Autodesk Inventor part; units mm, degrees
(part 2 of 3)
  line L1031 (-10.05, 26.35) -> (-10.15, 26.35)
  line L1032 (-10.15, 26.35) -> (-10.15, 26.05)
  line L1033 (-10.05, 26.05) -> (-10.05, 26.35)
  line L1034 (-9.175, 25.6738) -> (-9.175, 25.9738)
  line L1035 (-9.275, 25.9738) -> (-9.275, 25.6738)
  line L1036 (-9.275, 25.6738) -> (-9.175, 25.6738)
  line L1037 (-9.425, 25.6738) -> (-9.425, 25.9738)
  line L1038 (-9.525, 25.9738) -> (-9.525, 25.6738)
  line L1039 (-9.525, 25.6738) -> (-9.425, 25.6738)
  line L1040 (-9.425, 25.9738) -> (-9.525, 25.9738)
  line L1041 (-9.175, 25.9738) -> (-9.275, 25.9738)
  line L1042 (-8.675, 25.6738) -> (-8.675, 25.9738)
  line L1043 (-8.775, 25.9738) -> (-8.775, 25.6738)
  line L1044 (-8.675, 25.9738) -> (-8.775, 25.9738)
  line L1045 (-8.775, 25.6738) -> (-8.675, 25.6738)
  line L1046 (-8.925, 25.6738) -> (-8.925, 25.9738)
  line L1047 (-8.925, 25.9738) -> (-9.025, 25.9738)
  line L1048 (-9.025, 25.9738) -> (-9.025, 25.6738)
  line L1049 (-9.025, 25.6738) -> (-8.925, 25.6738)
  line L1050 (-8.175, 25.9738) -> (-8.275, 25.9738)
  line L1051 (-8.425, 25.9738) -> (-8.525, 25.9738)
  line L1052 (-8.175, 25.6738) -> (-8.175, 25.9738)
  line L1053 (-8.275, 25.9738) -> (-8.275, 25.6738)
  line L1054 (-8.275, 25.6738) -> (-8.175, 25.6738)
  line L1055 (-8.425, 25.6738) -> (-8.425, 25.9738)
  line L1056 (-8.525, 25.9738) -> (-8.525, 25.6738)
  line L1057 (-8.525, 25.6738) -> (-8.425, 25.6738)
  line L1058 (-7.775, 25.9738) -> (-7.775, 25.6738)
  line L1059 (-7.675, 25.9738) -> (-7.775, 25.9738)
  line L1060 (-7.775, 25.6738) -> (-7.675, 25.6738)
  line L1061 (-7.925, 25.6738) -> (-7.925, 25.9738)
  line L1062 (-8.025, 25.9738) -> (-8.025, 25.6738)
  line L1063 (-7.925, 25.9738) -> (-8.025, 25.9738)
  line L1064 (-8.025, 25.6738) -> (-7.925, 25.6738)
  line L1065 (-7.675, 25.6738) -> (-7.675, 25.9738)
  line L1066 (-7.425, 25.9738) -> (-7.525, 25.9738)
  line L1067 (-7.175, 25.9738) -> (-7.275, 25.9738)
  line L1068 (-7.525, 25.9738) -> (-7.525, 25.6738)
  line L1069 (-7.525, 25.6738) -> (-7.425, 25.6738)
  line L1070 (-7.425, 25.6738) -> (-7.425, 25.9738)
  line L1071 (-7.275, 25.9738) -> (-7.275, 25.6738)
  line L1072 (-7.275, 25.6738) -> (-7.175, 25.6738)
  line L1073 (-6.925, 25.9738) -> (-7.025, 25.9738)
  line L1074 (-7.025, 25.9738) -> (-7.025, 25.6738)
  line L1075 (-7.025, 25.6738) -> (-6.925, 25.6738)
  line L1076 (-6.925, 25.6738) -> (-6.925, 25.9738)
  line L1077 (-7.175, 25.6738) -> (-7.175, 25.9738)
  line L1078 (-5.775, 25.9738) -> (-5.775, 25.6738)
  line L1079 (-5.675, 25.9738) -> (-5.775, 25.9738)
  line L1080 (-5.775, 25.6738) -> (-5.675, 25.6738)
  line L1081 (-5.925, 25.6738) -> (-5.925, 25.9738)
  line L1082 (-6.025, 25.6738) -> (-5.925, 25.6738)
  line L1083 (-5.925, 25.9738) -> (-6.025, 25.9738)
  line L1084 (-6.025, 25.9738) -> (-6.025, 25.6738)
  line L1085 (-6.175, 25.6738) -> (-6.175, 25.9738)
  line L1086 (-6.275, 25.9738) -> (-6.275, 25.6738)
  line L1087 (-6.175, 25.9738) -> (-6.275, 25.9738)
  line L1088 (-6.275, 25.6738) -> (-6.175, 25.6738)
  line L1089 (-5.675, 25.6738) -> (-5.675, 25.9738)
  line L1090 (-5.425, 25.9738) -> (-5.525, 25.9738)
  line L1091 (-5.525, 25.9738) -> (-5.525, 25.6738)
  line L1092 (-5.525, 25.6738) -> (-5.425, 25.6738)
  line L1093 (-5.425, 25.6738) -> (-5.425, 25.9738)
  line L1094 (-5.275, 25.9738) -> (-5.275, 25.6738)
  line L1095 (-5.175, 25.6738) -> (-5.175, 25.9738)
  line L1096 (-5.275, 25.6738) -> (-5.175, 25.6738)
  line L1097 (-5.175, 25.9738) -> (-5.275, 25.9738)
  line L1098 (-4.675, 25.6738) -> (-4.675, 25.9738)
  line L1099 (-4.675, 25.9738) -> (-4.775, 25.9738)
  line L1100 (-4.775, 25.6738) -> (-4.675, 25.6738)
  line L1101 (-4.775, 25.9738) -> (-4.775, 25.6738)
  line L1102 (-4.925, 25.6738) -> (-4.925, 25.9738)
  line L1103 (-5.025, 25.9738) -> (-5.025, 25.6738)
  line L1104 (-5.025, 25.6738) -> (-4.925, 25.6738)
  line L1105 (-4.925, 25.9738) -> (-5.025, 25.9738)
  line L1106 (-4.175, 25.9738) -> (-4.275, 25.9738)
  line L1107 (-4.425, 25.9738) -> (-4.525, 25.9738)
  line L1108 (-4.525, 25.9738) -> (-4.525, 25.6738)
  line L1109 (-4.525, 25.6738) -> (-4.425, 25.6738)
  line L1110 (-4.425, 25.6738) -> (-4.425, 25.9738)
  line L1111 (-4.275, 25.9738) -> (-4.275, 25.6738)
  line L1112 (-4.175, 25.6738) -> (-4.175, 25.9738)
  line L1113 (-4.275, 25.6738) -> (-4.175, 25.6738)
  line L1114 (-3.55, 26.35) -> (-3.65, 26.35)
  line L1115 (-3.65, 26.35) -> (-3.65, 26.05)
  line L1116 (-3.65, 26.05) -> (-3.55, 26.05)
  line L1117 (-3.55, 26.05) -> (-3.55, 26.35)
  line L1118 (-3.425, 25.9738) -> (-3.525, 25.9738)
  line L1119 (-3.525, 25.9738) -> (-3.525, 25.6738)
  line L1120 (-3.525, 25.6738) -> (-3.425, 25.6738)
  line L1121 (-4.025, 25.9738) -> (-4.025, 25.6738)
  line L1122 (-3.925, 25.9738) -> (-4.025, 25.9738)
  line L1123 (-4.025, 25.6738) -> (-3.925, 25.6738)
  line L1124 (-3.925, 25.6738) -> (-3.925, 25.9738)
  line L1125 (-3.775, 25.9738) -> (-3.775, 25.6738)
  line L1126 (-3.675, 25.9738) -> (-3.775, 25.9738)
  line L1127 (-3.775, 25.6738) -> (-3.675, 25.6738)
  line L1128 (-3.675, 25.6738) -> (-3.675, 25.9738)
  line L1129 (-3.425, 25.6738) -> (-3.425, 25.9738)
  line L1130 (-6.425, 25.9738) -> (-6.525, 25.9738)
  line L1131 (-6.675, 25.9738) -> (-6.775, 25.9738)
  line L1132 (-6.425, 25.6738) -> (-6.425, 25.9738)
  line L1133 (-6.525, 25.9738) -> (-6.525, 25.6738)
  line L1134 (-6.675, 25.6738) -> (-6.675, 25.9738)
  line L1135 (-6.775, 25.9738) -> (-6.775, 25.6738)
  line L1136 (-6.775, 25.6738) -> (-6.675, 25.6738)
  line L1137 (-6.525, 25.6738) -> (-6.425, 25.6738)
  line L1138 (19.6272, 0) -> (-14.05, 0) construction
  line L1139 (-16.8, -26.05) -> (-16.8, -26.35)
  line L1140 (-16.7, -26.05) -> (-16.8, -26.05)
  line L1141 (-16.8, -26.35) -> (-16.7, -26.35)
  line L1142 (-16.7, -26.35) -> (-16.7, -26.05)
  line L1143 (-16.55, -26.05) -> (-16.55, -26.35)
  line L1144 (-16.55, -26.35) -> (-16.45, -26.35)
  line L1145 (-16.45, -26.05) -> (-16.55, -26.05)
  line L1146 (-16.45, -26.35) -> (-16.45, -26.05)
  line L1147 (-16.3, -26.05) -> (-16.3, -26.35)
  line L1148 (-16.2, -26.05) -> (-16.3, -26.05)
  line L1149 (-16.3, -26.35) -> (-16.2, -26.35)
  line L1150 (-16.05, -26.05) -> (-16.05, -26.35)
  line L1151 (-15.95, -26.05) -> (-16.05, -26.05)
  line L1152 (-15.95, -26.35) -> (-15.95, -26.05)
  line L1153 (-16.05, -26.35) -> (-15.95, -26.35)
  line L1154 (-15.8, -26.05) -> (-15.8, -26.35)
  line L1155 (-15.7, -26.05) -> (-15.8, -26.05)
  line L1156 (-15.7, -26.35) -> (-15.7, -26.05)
  line L1157 (-15.8, -26.35) -> (-15.7, -26.35)
  line L1158 (-16.2, -26.35) -> (-16.2, -26.05)
  line L1159 (-17.8, -26.35) -> (-17.7, -26.35)
  line L1160 (-17.7, -26.35) -> (-17.7, -26.05)
  line L1161 (-17.7, -26.05) -> (-17.8, -26.05)
  line L1162 (-17.8, -26.05) -> (-17.8, -26.35)
  line L1163 (-17.55, -26.35) -> (-17.45, -26.35)
  line L1164 (-17.45, -26.35) -> (-17.45, -26.05)
  line L1165 (-17.45, -26.05) -> (-17.55, -26.05)
  line L1166 (-17.55, -26.05) -> (-17.55, -26.35)
  line L1167 (-16.95, -26.35) -> (-16.95, -26.05)
  line L1168 (-17.05, -26.35) -> (-16.95, -26.35)
  line L1169 (-16.95, -26.05) -> (-17.05, -26.05)
  line L1170 (-17.05, -26.05) -> (-17.05, -26.35)
  line L1171 (-17.2, -26.35) -> (-17.2, -26.05)
  line L1172 (-17.2, -26.05) -> (-17.3, -26.05)
  line L1173 (-17.3, -26.05) -> (-17.3, -26.35)
  line L1174 (-17.3, -26.35) -> (-17.2, -26.35)
  line L1175 (-15.45, -26.05) -> (-15.55, -26.05)
  line L1176 (-15.45, -26.35) -> (-15.45, -26.05)
  line L1177 (-15.55, -26.35) -> (-15.45, -26.35)
  line L1178 (-15.3, -26.05) -> (-15.3, -26.35)
  line L1179 (-15.2, -26.05) -> (-15.3, -26.05)
  line L1180 (-15.3, -26.35) -> (-15.2, -26.35)
  line L1181 (-15.2, -26.35) -> (-15.2, -26.05)
  line L1182 (-15.55, -26.05) -> (-15.55, -26.35)
  line L1183 (-15.05, -26.05) -> (-15.05, -26.35)
  line L1184 (-14.95, -26.35) -> (-14.95, -26.05)
  line L1185 (-15.05, -26.35) -> (-14.95, -26.35)
  line L1186 (-14.8, -26.05) -> (-14.8, -26.35)
  line L1187 (-14.7, -26.35) -> (-14.7, -26.05)
  line L1188 (-14.8, -26.35) -> (-14.7, -26.35)
  line L1189 (-14.7, -26.05) -> (-14.8, -26.05)
  line L1190 (-14.95, -26.05) -> (-15.05, -26.05)
  line L1191 (-14.55, -26.05) -> (-14.55, -26.35)
  line L1192 (-14.45, -26.05) -> (-14.55, -26.05)
  line L1193 (-14.45, -26.35) -> (-14.45, -26.05)
  line L1194 (-14.3, -26.05) -> (-14.3, -26.35)
  line L1195 (-14.2, -26.05) -> (-14.3, -26.05)
  line L1196 (-14.2, -26.35) -> (-14.2, -26.05)
  line L1197 (-14.3, -26.35) -> (-14.2, -26.35)
  line L1198 (-14.55, -26.35) -> (-14.45, -26.35)
  line L1199 (-14.05, -26.05) -> (-14.05, -26.35)
  line L1200 (-13.95, -26.05) -> (-14.05, -26.05)
  line L1201 (-13.95, -26.35) -> (-13.95, -26.05)
  line L1202 (-14.05, -26.35) -> (-13.95, -26.35)
  line L1203 (-13.8, -26.05) -> (-13.8, -26.35)
  line L1204 (-13.7, -26.35) -> (-13.7, -26.05)
  line L1205 (-13.8, -26.35) -> (-13.7, -26.35)
  line L1206 (-13.7, -26.05) -> (-13.8, -26.05)
  line L1207 (-13.55, -26.05) -> (-13.55, -26.35)
  line L1208 (-13.45, -26.05) -> (-13.55, -26.05)
  line L1209 (-13.55, -26.35) -> (-13.45, -26.35)
  line L1210 (-13.3, -26.05) -> (-13.3, -26.35)
  line L1211 (-13.2, -26.05) -> (-13.3, -26.05)
  line L1212 (-13.3, -26.35) -> (-13.2, -26.35)
  line L1213 (-13.2, -26.35) -> (-13.2, -26.05)
  line L1214 (-13.45, -26.35) -> (-13.45, -26.05)
  line L1215 (-13.05, -26.05) -> (-13.05, -26.35)
  line L1216 (-12.95, -26.05) -> (-13.05, -26.05)
  line L1217 (-13.05, -26.35) -> (-12.95, -26.35)
  line L1218 (-12.95, -26.35) -> (-12.95, -26.05)
  line L1219 (-12.8, -26.05) -> (-12.8, -26.35)
  line L1220 (-12.7, -26.35) -> (-12.7, -26.05)
  line L1221 (-12.8, -26.35) -> (-12.7, -26.35)
  line L1222 (-12.7, -26.05) -> (-12.8, -26.05)
  line L1223 (-12.55, -26.05) -> (-12.55, -26.35)
  line L1224 (-12.45, -26.05) -> (-12.55, -26.05)
  line L1225 (-12.55, -26.35) -> (-12.45, -26.35)
  line L1226 (-12.45, -26.35) -> (-12.45, -26.05)
  line L1227 (-12.3, -26.05) -> (-12.3, -26.35)
  line L1228 (-12.2, -26.05) -> (-12.3, -26.05)
  line L1229 (-12.2, -26.35) -> (-12.2, -26.05)
  line L1230 (-12.3, -26.35) -> (-12.2, -26.35)
  line L1231 (-12.05, -26.05) -> (-12.05, -26.35)
  line L1232 (-11.95, -26.05) -> (-12.05, -26.05)
  line L1233 (-12.05, -26.35) -> (-11.95, -26.35)
  line L1234 (-11.95, -26.35) -> (-11.95, -26.05)
  line L1235 (-11.7, -26.05) -> (-11.8, -26.05)
  line L1236 (-11.7, -26.35) -> (-11.7, -26.05)
  line L1237 (-11.8, -26.35) -> (-11.7, -26.35)
  line L1238 (-11.8, -26.05) -> (-11.8, -26.35)
  line L1239 (-7.925, -25.9738) -> (-7.825, -25.9738)
  line L1240 (-7.675, -25.9738) -> (-7.575, -25.9738)
  line L1241 (-7.925, -25.6738) -> (-7.925, -25.9738)
  line L1242 (-7.825, -25.6738) -> (-7.925, -25.6738)
  line L1243 (-7.825, -25.9738) -> (-7.825, -25.6738)
  line L1244 (-7.675, -25.6738) -> (-7.675, -25.9738)
  line L1245 (-7.575, -25.9738) -> (-7.575, -25.6738)
  line L1246 (-7.575, -25.6738) -> (-7.675, -25.6738)
  line L1247 (-8.425, -25.6738) -> (-8.425, -25.9738)
  line L1248 (-8.425, -25.9738) -> (-8.325, -25.9738)
  line L1249 (-8.325, -25.6738) -> (-8.425, -25.6738)
  line L1250 (-8.325, -25.9738) -> (-8.325, -25.6738)
  line L1251 (-8.175, -25.6738) -> (-8.175, -25.9738)
  line L1252 (-8.075, -25.9738) -> (-8.075, -25.6738)
  line L1253 (-8.075, -25.6738) -> (-8.175, -25.6738)
  line L1254 (-8.175, -25.9738) -> (-8.075, -25.9738)
  line L1255 (-8.55, -26.35) -> (-8.45, -26.35)
  line L1256 (-8.45, -26.35) -> (-8.45, -26.05)
  line L1257 (-8.45, -26.05) -> (-8.55, -26.05)
  line L1258 (-8.55, -26.05) -> (-8.55, -26.35)
  line L1259 (-8.3, -26.35) -> (-8.2, -26.35)
  line L1260 (-8.2, -26.35) -> (-8.2, -26.05)
  line L1261 (-8.2, -26.05) -> (-8.3, -26.05)
  line L1262 (-7.95, -26.05) -> (-8.05, -26.05)
  line L1263 (-7.7, -26.35) -> (-7.7, -26.05)
  line L1264 (-7.8, -26.35) -> (-7.7, -26.35)
  line L1265 (-7.8, -26.05) -> (-7.8, -26.35)
  line L1266 (-7.95, -26.35) -> (-7.95, -26.05)
  line L1267 (-8.05, -26.35) -> (-7.95, -26.35)
  line L1268 (-8.05, -26.05) -> (-8.05, -26.35)
  line L1269 (-8.3, -26.05) -> (-8.3, -26.35)
  line L1270 (-7.7, -26.05) -> (-7.8, -26.05)
  line L1271 (-9.05, -26.05) -> (-9.05, -26.35)
  line L1272 (-8.95, -26.05) -> (-9.05, -26.05)
  line L1273 (-9.05, -26.35) -> (-8.95, -26.35)
  line L1274 (-8.95, -26.35) -> (-8.95, -26.05)
  line L1275 (-8.925, -25.9738) -> (-8.825, -25.9738)
  line L1276 (-8.7, -26.05) -> (-8.8, -26.05)
  line L1277 (-8.8, -26.35) -> (-8.7, -26.35)
  line L1278 (-8.7, -26.35) -> (-8.7, -26.05)
  line L1279 (-8.925, -25.6738) -> (-8.925, -25.9738)
  line L1280 (-8.825, -25.6738) -> (-8.925, -25.6738)
  line L1281 (-8.675, -25.9738) -> (-8.575, -25.9738)
  line L1282 (-8.825, -25.9738) -> (-8.825, -25.6738)
  line L1283 (-8.675, -25.6738) -> (-8.675, -25.9738)
  line L1284 (-8.575, -25.9738) -> (-8.575, -25.6738)
  line L1285 (-8.575, -25.6738) -> (-8.675, -25.6738)
  line L1286 (-8.8, -26.05) -> (-8.8, -26.35)
  line L1287 (-9.425, -25.6738) -> (-9.425, -25.9738)
  line L1288 (-9.325, -25.6738) -> (-9.425, -25.6738)
  line L1289 (-9.425, -25.9738) -> (-9.325, -25.9738)
  line L1290 (-9.325, -25.9738) -> (-9.325, -25.6738)
  line L1291 (-9.175, -25.6738) -> (-9.175, -25.9738)
  line L1292 (-9.075, -25.9738) -> (-9.075, -25.6738)
  line L1293 (-9.175, -25.9738) -> (-9.075, -25.9738)
  line L1294 (-9.075, -25.6738) -> (-9.175, -25.6738)
  line L1295 (-18.3, -26.35) -> (-18.2, -26.35)
  line L1296 (-18.2, -26.35) -> (-18.2, -26.05)
  line L1297 (-18.2, -26.05) -> (-18.3, -26.05)
  line L1298 (-18.3, -26.05) -> (-18.3, -26.35)
  line L1299 (-10.05, -26.05) -> (-10.05, -26.35)
  line L1300 (-9.95, -26.05) -> (-10.05, -26.05)
  line L1301 (-10.05, -26.35) -> (-9.95, -26.35)
  line L1302 (-9.95, -26.35) -> (-9.95, -26.05)
  line L1303 (-9.8, -26.05) -> (-9.8, -26.35)
  line L1304 (-9.7, -26.05) -> (-9.8, -26.05)
  line L1305 (-9.8, -26.35) -> (-9.7, -26.35)
  line L1306 (-9.7, -26.35) -> (-9.7, -26.05)
  line L1307 (-10.55, -26.05) -> (-10.55, -26.35)
  line L1308 (-10.45, -26.05) -> (-10.55, -26.05)
  line L1309 (-10.55, -26.35) -> (-10.45, -26.35)
  line L1310 (-10.45, -26.35) -> (-10.45, -26.05)
  line L1311 (-10.3, -26.05) -> (-10.3, -26.35)
  line L1312 (-10.2, -26.05) -> (-10.3, -26.05)
  line L1313 (-10.2, -26.35) -> (-10.2, -26.05)
  line L1314 (-10.3, -26.35) -> (-10.2, -26.35)
  line L1315 (-11.05, -26.05) -> (-11.05, -26.35)
  line L1316 (-10.95, -26.05) -> (-11.05, -26.05)
  line L1317 (-11.05, -26.35) -> (-10.95, -26.35)
  line L1318 (-10.95, -26.35) -> (-10.95, -26.05)
  line L1319 (-10.8, -26.05) -> (-10.8, -26.35)
  line L1320 (-10.7, -26.35) -> (-10.7, -26.05)
  line L1321 (-10.8, -26.35) -> (-10.7, -26.35)
  line L1322 (-10.7, -26.05) -> (-10.8, -26.05)
  line L1323 (-11.55, -26.05) -> (-11.55, -26.35)
  line L1324 (-11.45, -26.05) -> (-11.55, -26.05)
  line L1325 (-11.55, -26.35) -> (-11.45, -26.35)
  line L1326 (-11.45, -26.35) -> (-11.45, -26.05)
  line L1327 (-11.3, -26.05) -> (-11.3, -26.35)
  line L1328 (-11.2, -26.35) -> (-11.2, -26.05)
  line L1329 (-11.3, -26.35) -> (-11.2, -26.35)
  line L1330 (-11.2, -26.05) -> (-11.3, -26.05)
  line L1331 (-18.05, -26.35) -> (-17.95, -26.35)
  line L1332 (-17.95, -26.35) -> (-17.95, -26.05)
  line L1333 (-17.95, -26.05) -> (-18.05, -26.05)
  line L1334 (-18.05, -26.05) -> (-18.05, -26.35)
  line L1335 (-18.175, -25.9738) -> (-18.075, -25.9738)
  line L1336 (-18.075, -25.9738) -> (-18.075, -25.6738)
  line L1337 (-17.575, -25.9738) -> (-17.575, -25.6738)
  line L1338 (-17.675, -25.9738) -> (-17.575, -25.9738)
  line L1339 (-17.575, -25.6738) -> (-17.675, -25.6738)
  line L1340 (-17.825, -25.9738) -> (-17.825, -25.6738)
  line L1341 (-17.825, -25.6738) -> (-17.925, -25.6738)
  line L1342 (-17.925, -25.6738) -> (-17.925, -25.9738)
  line L1343 (-18.075, -25.6738) -> (-18.175, -25.6738)
  line L1344 (-18.175, -25.6738) -> (-18.175, -25.9738)
  line L1345 (-17.925, -25.9738) -> (-17.825, -25.9738)
  line L1346 (-9.55, -26.05) -> (-9.55, -26.35)
  line L1347 (-9.45, -26.05) -> (-9.55, -26.05)
  line L1348 (-9.55, -26.35) -> (-9.45, -26.35)
  line L1349 (-9.45, -26.35) -> (-9.45, -26.05)
  line L1350 (-9.3, -26.05) -> (-9.3, -26.35)
  line L1351 (-9.2, -26.05) -> (-9.3, -26.05)
  line L1352 (-9.2, -26.35) -> (-9.2, -26.05)
  line L1353 (-9.3, -26.35) -> (-9.2, -26.35)
  line L1354 (-7.425, -25.6738) -> (-7.425, -25.9738)
  line L1355 (-7.425, -25.9738) -> (-7.325, -25.9738)
  line L1356 (-7.325, -25.6738) -> (-7.425, -25.6738)
  line L1357 (-7.325, -25.9738) -> (-7.325, -25.6738)
  line L1358 (-7.175, -25.6738) -> (-7.175, -25.9738)
  line L1359 (-7.075, -25.9738) -> (-7.075, -25.6738)
  line L1360 (-7.075, -25.6738) -> (-7.175, -25.6738)
  line L1361 (-7.175, -25.9738) -> (-7.075, -25.9738)
  line L1362 (-6.925, -25.9738) -> (-6.825, -25.9738)
  line L1363 (-6.675, -25.9738) -> (-6.575, -25.9738)
  line L1364 (-6.925, -25.6738) -> (-6.925, -25.9738)
  line L1365 (-6.825, -25.6738) -> (-6.925, -25.6738)
  line L1366 (-6.825, -25.9738) -> (-6.825, -25.6738)
  line L1367 (-6.675, -25.6738) -> (-6.675, -25.9738)
  line L1368 (-6.575, -25.9738) -> (-6.575, -25.6738)
  line L1369 (-6.575, -25.6738) -> (-6.675, -25.6738)
  line L1370 (-6.425, -25.6738) -> (-6.425, -25.9738)
  line L1371 (-6.425, -25.9738) -> (-6.325, -25.9738)
  line L1372 (-6.325, -25.6738) -> (-6.425, -25.6738)
  line L1373 (-6.325, -25.9738) -> (-6.325, -25.6738)
  line L1374 (-6.175, -25.6738) -> (-6.175, -25.9738)
  line L1375 (-6.175, -25.9738) -> (-6.075, -25.9738)
  line L1376 (-6.075, -25.9738) -> (-6.075, -25.6738)
  line L1377 (-6.075, -25.6738) -> (-6.175, -25.6738)
  line L1378 (-5.925, -25.6738) -> (-5.925, -25.9738)
  line L1379 (-6.55, -26.35) -> (-6.45, -26.35)
  line L1380 (-6.45, -26.35) -> (-6.45, -26.05)
  line L1381 (-6.45, -26.05) -> (-6.55, -26.05)
  line L1382 (-5.95, -26.05) -> (-6.05, -26.05)
  line L1383 (-5.7, -26.35) -> (-5.7, -26.05)
  line L1384 (-5.8, -26.35) -> (-5.7, -26.35)
  line L1385 (-5.8, -26.05) -> (-5.8, -26.35)
  line L1386 (-6.2, -26.05) -> (-6.3, -26.05)
  line L1387 (-5.95, -26.35) -> (-5.95, -26.05)
  line L1388 (-6.05, -26.05) -> (-6.05, -26.35)
  line L1389 (-6.2, -26.35) -> (-6.2, -26.05)
  line L1390 (-6.3, -26.35) -> (-6.2, -26.35)
  line L1391 (-6.3, -26.05) -> (-6.3, -26.35)
  line L1392 (-6.55, -26.05) -> (-6.55, -26.35)
  line L1393 (-6.05, -26.35) -> (-5.95, -26.35)
  line L1394 (-5.925, -25.9738) -> (-5.825, -25.9738)
  line L1395 (-5.7, -26.05) -> (-5.8, -26.05)
  line L1396 (-5.825, -25.6738) -> (-5.925, -25.6738)
  line L1397 (-5.825, -25.9738) -> (-5.825, -25.6738)
  line L1398 (-5.675, -25.6738) -> (-5.675, -25.9738)
  line L1399 (-5.675, -25.9738) -> (-5.575, -25.9738)
  line L1400 (-5.575, -25.6738) -> (-5.675, -25.6738)
  line L1401 (-5.575, -25.9738) -> (-5.575, -25.6738)
  line L1402 (-5.425, -25.6738) -> (-5.425, -25.9738)
  line L1403 (-5.325, -25.6738) -> (-5.425, -25.6738)
  line L1404 (-5.325, -25.9738) -> (-5.325, -25.6738)
  line L1405 (-5.425, -25.9738) -> (-5.325, -25.9738)
  line L1406 (-5.175, -25.9738) -> (-5.075, -25.9738)
  line L1407 (-4.925, -25.9738) -> (-4.825, -25.9738)
  line L1408 (-4.825, -25.9738) -> (-4.825, -25.6738)
  line L1409 (-4.925, -25.6738) -> (-4.925, -25.9738)
  line L1410 (-4.825, -25.6738) -> (-4.925, -25.6738)
  line L1411 (-5.075, -25.9738) -> (-5.075, -25.6738)
  line L1412 (-5.175, -25.6738) -> (-5.175, -25.9738)
  line L1413 (-5.075, -25.6738) -> (-5.175, -25.6738)
  line L1414 (-5.55, -26.35) -> (-5.45, -26.35)
  line L1415 (-5.45, -26.35) -> (-5.45, -26.05)
  line L1416 (-5.45, -26.05) -> (-5.55, -26.05)
  line L1417 (-5.55, -26.05) -> (-5.55, -26.35)
  line L1418 (-5.3, -26.35) -> (-5.2, -26.35)
  line L1419 (-5.2, -26.35) -> (-5.2, -26.05)
  line L1420 (-5.2, -26.05) -> (-5.3, -26.05)
  line L1421 (-4.95, -26.05) -> (-5.05, -26.05)
  line L1422 (-4.7, -26.05) -> (-4.8, -26.05)
  line L1423 (-5.3, -26.05) -> (-5.3, -26.35)
  line L1424 (-5.05, -26.35) -> (-4.95, -26.35)
  line L1425 (-5.05, -26.05) -> (-5.05, -26.35)
  line L1426 (-4.95, -26.35) -> (-4.95, -26.05)
  line L1427 (-4.8, -26.05) -> (-4.8, -26.35)
  line L1428 (-4.7, -26.35) -> (-4.7, -26.05)
  line L1429 (-4.8, -26.35) -> (-4.7, -26.35)
  line L1430 (-4.675, -25.6738) -> (-4.675, -25.9738)
  line L1431 (-4.575, -25.9738) -> (-4.575, -25.6738)
  line L1432 (-4.675, -25.9738) -> (-4.575, -25.9738)
  line L1433 (-4.425, -25.6738) -> (-4.425, -25.9738)
  line L1434 (-4.325, -25.9738) -> (-4.325, -25.6738)
  line L1435 (-4.425, -25.9738) -> (-4.325, -25.9738)
  line L1436 (-4.325, -25.6738) -> (-4.425, -25.6738)
  line L1437 (-4.575, -25.6738) -> (-4.675, -25.6738)
  line L1438 (-4.175, -25.9738) -> (-4.075, -25.9738)
  line L1439 (-3.925, -25.9738) -> (-3.825, -25.9738)
  line L1440 (-3.825, -25.9738) -> (-3.825, -25.6738)
  line L1441 (-3.825, -25.6738) -> (-3.925, -25.6738)
  line L1442 (-4.075, -25.9738) -> (-4.075, -25.6738)
  line L1443 (-4.175, -25.6738) -> (-4.175, -25.9738)
  line L1444 (-4.075, -25.6738) -> (-4.175, -25.6738)
  line L1445 (-3.925, -25.6738) -> (-3.925, -25.9738)
  line L1446 (-4.55, -26.35) -> (-4.45, -26.35)
  line L1447 (-4.45, -26.35) -> (-4.45, -26.05)
  line L1448 (-4.45, -26.05) -> (-4.55, -26.05)
  line L1449 (-4.55, -26.05) -> (-4.55, -26.35)
  line L1450 (-4.3, -26.35) -> (-4.2, -26.35)
  line L1451 (-4.2, -26.35) -> (-4.2, -26.05)
  line L1452 (-4.2, -26.05) -> (-4.3, -26.05)
  line L1453 (-3.95, -26.05) -> (-4.05, -26.05)
  line L1454 (-3.7, -26.05) -> (-3.8, -26.05)
  line L1455 (-4.3, -26.05) -> (-4.3, -26.35)
  line L1456 (-4.05, -26.35) -> (-3.95, -26.35)
  line L1457 (-4.05, -26.05) -> (-4.05, -26.35)
  line L1458 (-3.95, -26.35) -> (-3.95, -26.05)
  line L1459 (-3.8, -26.05) -> (-3.8, -26.35)
  line L1460 (-3.8, -26.35) -> (-3.7, -26.35)
  line L1461 (-3.7, -26.35) -> (-3.7, -26.05)
  line L1462 (-3.675, -25.6738) -> (-3.675, -25.9738)
  line L1463 (-3.575, -25.9738) -> (-3.575, -25.6738)
  line L1464 (-3.675, -25.9738) -> (-3.575, -25.9738)
  line L1465 (-3.575, -25.6738) -> (-3.675, -25.6738)
  line L1466 (-3.425, -25.6738) -> (-3.425, -25.9738)
  line L1467 (-3.325, -25.9738) -> (-3.325, -25.6738)
  line L1468 (-3.325, -25.6738) -> (-3.425, -25.6738)
  line L1469 (-3.425, -25.9738) -> (-3.325, -25.9738)
  line L1470 (-3.175, -25.9738) -> (-3.075, -25.9738)
  line L1471 (-2.925, -25.9738) -> (-2.825, -25.9738)
  line L1472 (-2.825, -25.9738) -> (-2.825, -25.6738)
  line L1473 (-2.825, -25.6738) -> (-2.925, -25.6738)
  line L1474 (-2.925, -25.6738) -> (-2.925, -25.9738)
  line L1475 (-3.075, -25.9738) -> (-3.075, -25.6738)
  line L1476 (-3.175, -25.6738) -> (-3.175, -25.9738)
  line L1477 (-3.075, -25.6738) -> (-3.175, -25.6738)
  line L1478 (-3.55, -26.35) -> (-3.45, -26.35)
  line L1479 (-3.45, -26.35) -> (-3.45, -26.05)
  line L1480 (-3.45, -26.05) -> (-3.55, -26.05)
  line L1481 (-3.55, -26.05) -> (-3.55, -26.35)
  line L1482 (-3.3, -26.35) -> (-3.2, -26.35)
  line L1483 (-3.2, -26.35) -> (-3.2, -26.05)
  line L1484 (-3.2, -26.05) -> (-3.3, -26.05)
  line L1485 (-2.95, -26.05) -> (-3.05, -26.05)
  line L1486 (-2.7, -26.05) -> (-2.8, -26.05)
  line L1487 (-3.3, -26.05) -> (-3.3, -26.35)
  line L1488 (-3.05, -26.35) -> (-2.95, -26.35)
  line L1489 (-3.05, -26.05) -> (-3.05, -26.35)
  line L1490 (-2.95, -26.35) -> (-2.95, -26.05)
  line L1491 (-2.8, -26.05) -> (-2.8, -26.35)
  line L1492 (-2.7, -26.35) -> (-2.7, -26.05)
  line L1493 (-2.8, -26.35) -> (-2.7, -26.35)
  line L1494 (-2.675, -25.6738) -> (-2.675, -25.9738)
  line L1495 (-2.675, -25.9738) -> (-2.575, -25.9738)
  line L1496 (-2.575, -25.6738) -> (-2.675, -25.6738)
  line L1497 (-2.575, -25.9738) -> (-2.575, -25.6738)
  line L1498 (-2.425, -25.6738) -> (-2.425, -25.9738)
  line L1499 (-2.425, -25.9738) -> (-2.325, -25.9738)
  line L1500 (-2.325, -25.6738) -> (-2.425, -25.6738)
  line L1501 (-2.325, -25.9738) -> (-2.325, -25.6738)
  line L1502 (-2.175, -25.6738) -> (-2.175, -25.9738)
  line L1503 (-2.075, -25.9738) -> (-2.075, -25.6738)
  line L1504 (-2.175, -25.9738) -> (-2.075, -25.9738)
  line L1505 (-2.075, -25.6738) -> (-2.175, -25.6738)
  line L1506 (-2.55, -26.35) -> (-2.45, -26.35)
  line L1507 (-2.45, -26.35) -> (-2.45, -26.05)
  line L1508 (-2.45, -26.05) -> (-2.55, -26.05)
  line L1509 (-2.55, -26.05) -> (-2.55, -26.35)
  line L1510 (-2.3, -26.35) -> (-2.2, -26.35)
  line L1511 (-2.2, -26.35) -> (-2.2, -26.05)
  line L1512 (-2.2, -26.05) -> (-2.3, -26.05)
  line L1513 (-1.7, -26.05) -> (-1.8, -26.05)
  line L1514 (-1.95, -26.05) -> (-2.05, -26.05)
  line L1515 (-1.8, -26.35) -> (-1.7, -26.35)
  line L1516 (-1.7, -26.35) -> (-1.7, -26.05)
  line L1517 (-1.8, -26.05) -> (-1.8, -26.35)
  line L1518 (-1.95, -26.35) -> (-1.95, -26.05)
  line L1519 (-2.05, -26.35) -> (-1.95, -26.35)
  line L1520 (-2.3, -26.05) -> (-2.3, -26.35)
  line L1521 (-2.05, -26.05) -> (-2.05, -26.35)
  line L1522 (-1.925, -25.9738) -> (-1.825, -25.9738)
  line L1523 (-1.925, -25.6738) -> (-1.925, -25.9738)
  line L1524 (-1.825, -25.6738) -> (-1.925, -25.6738)
  line L1525 (-1.675, -25.9738) -> (-1.575, -25.9738)
  line L1526 (-1.825, -25.9738) -> (-1.825, -25.6738)
  line L1527 (-1.675, -25.6738) -> (-1.675, -25.9738)
  line L1528 (-1.575, -25.9738) -> (-1.575, -25.6738)
  line L1529 (-1.575, -25.6738) -> (-1.675, -25.6738)
  line L1530 (-1.425, -25.6738) -> (-1.425, -25.9738)
  line L1531 (-1.325, -25.6738) -> (-1.425, -25.6738)
  line L1532 (-1.425, -25.9738) -> (-1.325, -25.9738)
  line L1533 (-1.325, -25.9738) -> (-1.325, -25.6738)
  line L1534 (-1.175, -25.6738) -> (-1.175, -25.9738)
  line L1535 (-1.075, -25.9738) -> (-1.075, -25.6738)
  line L1536 (-1.175, -25.9738) -> (-1.075, -25.9738)
  line L1537 (-1.075, -25.6738) -> (-1.175, -25.6738)
  line L1538 (-1.55, -26.35) -> (-1.45, -26.35)
  line L1539 (-1.45, -26.35) -> (-1.45, -26.05)
  line L1540 (-1.45, -26.05) -> (-1.55, -26.05)
  line L1541 (-1.55, -26.05) -> (-1.55, -26.35)
  line L1542 (-1.3, -26.35) -> (-1.2, -26.35)
  line L1543 (-1.2, -26.35) -> (-1.2, -26.05)
  line L1544 (-1.2, -26.05) -> (-1.3, -26.05)
  line L1545 (-0.7, -26.05) -> (-0.8, -26.05)
  line L1546 (-0.8, -26.35) -> (-0.7, -26.35)
  line L1547 (-0.7, -26.35) -> (-0.7, -26.05)
  line L1548 (-0.8, -26.05) -> (-0.8, -26.35)
  line L1549 (-0.95, -26.35) -> (-0.95, -26.05)
  line L1550 (-1.05, -26.35) -> (-0.95, -26.35)
  line L1551 (-1.05, -26.05) -> (-1.05, -26.35)
  line L1552 (-1.3, -26.05) -> (-1.3, -26.35)
  line L1553 (-0.95, -26.05) -> (-1.05, -26.05)
  line L1554 (-0.925, -25.9738) -> (-0.825, -25.9738)
  line L1555 (-0.925, -25.6738) -> (-0.925, -25.9738)
  line L1556 (-0.825, -25.6738) -> (-0.925, -25.6738)
  line L1557 (-0.675, -25.9738) -> (-0.575, -25.9738)
  line L1558 (-0.675, -25.6738) -> (-0.675, -25.9738)
  line L1559 (-0.575, -25.9738) -> (-0.575, -25.6738)
  line L1560 (-0.575, -25.6738) -> (-0.675, -25.6738)
  line L1561 (-0.825, -25.9738) -> (-0.825, -25.6738)
  line L1562 (-7.55, -26.35) -> (-7.45, -26.35)
  line L1563 (-7.45, -26.35) -> (-7.45, -26.05)
  line L1564 (-7.45, -26.05) -> (-7.55, -26.05)
  line L1565 (-7.55, -26.05) -> (-7.55, -26.35)
  line L1566 (-7.3, -26.35) -> (-7.2, -26.35)
  line L1567 (-7.2, -26.35) -> (-7.2, -26.05)
  line L1568 (-7.2, -26.05) -> (-7.3, -26.05)
  line L1569 (-6.7, -26.05) -> (-6.8, -26.05)
  line L1570 (-6.95, -26.05) -> (-7.05, -26.05)
  line L1571 (-6.8, -26.35) -> (-6.7, -26.35)
  line L1572 (-6.8, -26.05) -> (-6.8, -26.35)
  line L1573 (-6.95, -26.35) -> (-6.95, -26.05)
  line L1574 (-7.05, -26.35) -> (-6.95, -26.35)
  line L1575 (-7.05, -26.05) -> (-7.05, -26.35)
  line L1576 (-7.3, -26.05) -> (-7.3, -26.35)
  line L1577 (-6.7, -26.35) -> (-6.7, -26.05)
  line L1578 (-9.925, -25.6738) -> (-9.925, -25.9738)
  line L1579 (-9.925, -25.9738) -> (-9.825, -25.9738)
  line L1580 (-9.825, -25.6738) -> (-9.925, -25.6738)
  line L1581 (-9.825, -25.9738) -> (-9.825, -25.6738)
  line L1582 (-9.675, -25.6738) -> (-9.675, -25.9738)
  line L1583 (-9.575, -25.9738) -> (-9.575, -25.6738)
  line L1584 (-9.675, -25.9738) -> (-9.575, -25.9738)
  line L1585 (-9.575, -25.6738) -> (-9.675, -25.6738)
  line L1586 (-10.425, -25.6738) -> (-10.425, -25.9738)
  line L1587 (-10.425, -25.9738) -> (-10.325, -25.9738)
  line L1588 (-10.325, -25.6738) -> (-10.425, -25.6738)
  line L1589 (-10.175, -25.6738) -> (-10.175, -25.9738)
  line L1590 (-10.075, -25.9738) -> (-10.075, -25.6738)
  line L1591 (-10.175, -25.9738) -> (-10.075, -25.9738)
  line L1592 (-10.075, -25.6738) -> (-10.175, -25.6738)
  line L1593 (-10.325, -25.9738) -> (-10.325, -25.6738)
  line L1594 (-10.925, -25.6738) -> (-10.925, -25.9738)
  line L1595 (-10.925, -25.9738) -> (-10.825, -25.9738)
  line L1596 (-10.825, -25.6738) -> (-10.925, -25.6738)
  line L1597 (-10.825, -25.9738) -> (-10.825, -25.6738)
  line L1598 (-10.675, -25.6738) -> (-10.675, -25.9738)
  line L1599 (-10.575, -25.9738) -> (-10.575, -25.6738)
  line L1600 (-10.575, -25.6738) -> (-10.675, -25.6738)
  line L1601 (-10.675, -25.9738) -> (-10.575, -25.9738)
  line L1602 (-11.425, -25.6738) -> (-11.425, -25.9738)
  line L1603 (-11.325, -25.9738) -> (-11.325, -25.6738)
  line L1604 (-11.325, -25.6738) -> (-11.425, -25.6738)
  line L1605 (-11.175, -25.6738) -> (-11.175, -25.9738)
  line L1606 (-11.075, -25.9738) -> (-11.075, -25.6738)
  line L1607 (-11.075, -25.6738) -> (-11.175, -25.6738)
  line L1608 (-11.175, -25.9738) -> (-11.075, -25.9738)
  line L1609 (-11.425, -25.9738) -> (-11.325, -25.9738)
  line L1610 (-11.925, -25.6738) -> (-11.925, -25.9738)
  line L1611 (-11.825, -25.9738) -> (-11.825, -25.6738)
  line L1612 (-11.925, -25.9738) -> (-11.825, -25.9738)
  line L1613 (-11.825, -25.6738) -> (-11.925, -25.6738)
  line L1614 (-11.675, -25.6738) -> (-11.675, -25.9738)
  line L1615 (-11.675, -25.9738) -> (-11.575, -25.9738)
  line L1616 (-11.575, -25.9738) -> (-11.575, -25.6738)
  line L1617 (-11.575, -25.6738) -> (-11.675, -25.6738)
  line L1618 (-12.425, -25.6738) -> (-12.425, -25.9738)
  line L1619 (-12.325, -25.9738) -> (-12.325, -25.6738)
  line L1620 (-12.425, -25.9738) -> (-12.325, -25.9738)
  line L1621 (-12.175, -25.6738) -> (-12.175, -25.9738)
  line L1622 (-12.075, -25.9738) -> (-12.075, -25.6738)
  line L1623 (-12.175, -25.9738) -> (-12.075, -25.9738)
  line L1624 (-12.075, -25.6738) -> (-12.175, -25.6738)
  line L1625 (-12.325, -25.6738) -> (-12.425, -25.6738)
  line L1626 (-12.825, -25.9738) -> (-12.825, -25.6738)
  line L1627 (-12.925, -25.9738) -> (-12.825, -25.9738)
  line L1628 (-12.825, -25.6738) -> (-12.925, -25.6738)
  line L1629 (-12.675, -25.6738) -> (-12.675, -25.9738)
  line L1630 (-12.575, -25.9738) -> (-12.575, -25.6738)
  line L1631 (-12.675, -25.9738) -> (-12.575, -25.9738)
  line L1632 (-12.575, -25.6738) -> (-12.675, -25.6738)
  line L1633 (-12.925, -25.6738) -> (-12.925, -25.9738)
  line L1634 (-13.575, -25.9738) -> (-13.575, -25.6738)
  line L1635 (-13.675, -25.9738) -> (-13.575, -25.9738)
  line L1636 (-13.575, -25.6738) -> (-13.675, -25.6738)
  line L1637 (-13.425, -25.6738) -> (-13.425, -25.9738)
  line L1638 (-13.325, -25.9738) -> (-13.325, -25.6738)
  line L1639 (-13.425, -25.9738) -> (-13.325, -25.9738)
  line L1640 (-13.325, -25.6738) -> (-13.425, -25.6738)
  line L1641 (-13.175, -25.6738) -> (-13.175, -25.9738)
  line L1642 (-13.075, -25.9738) -> (-13.075, -25.6738)
  line L1643 (-13.075, -25.6738) -> (-13.175, -25.6738)
  line L1644 (-13.175, -25.9738) -> (-13.075, -25.9738)
  line L1645 (-13.675, -25.6738) -> (-13.675, -25.9738)
  line L1646 (-14.825, -25.9738) -> (-14.825, -25.6738)
  line L1647 (-14.925, -25.9738) -> (-14.825, -25.9738)
  line L1648 (-14.825, -25.6738) -> (-14.925, -25.6738)
  line L1649 (-14.675, -25.6738) -> (-14.675, -25.9738)
  line L1650 (-14.575, -25.6738) -> (-14.675, -25.6738)
  line L1651 (-14.675, -25.9738) -> (-14.575, -25.9738)
  line L1652 (-14.575, -25.9738) -> (-14.575, -25.6738)
  line L1653 (-14.425, -25.6738) -> (-14.425, -25.9738)
  line L1654 (-14.325, -25.9738) -> (-14.325, -25.6738)
  line L1655 (-14.425, -25.9738) -> (-14.325, -25.9738)
  line L1656 (-14.325, -25.6738) -> (-14.425, -25.6738)
  line L1657 (-14.925, -25.6738) -> (-14.925, -25.9738)
  line L1658 (-15.425, -25.6738) -> (-15.425, -25.9738)
  line L1659 (-15.425, -25.9738) -> (-15.325, -25.9738)
  line L1660 (-15.325, -25.6738) -> (-15.425, -25.6738)
  line L1661 (-15.325, -25.9738) -> (-15.325, -25.6738)
  line L1662 (-15.175, -25.6738) -> (-15.175, -25.9738)
  line L1663 (-15.075, -25.9738) -> (-15.075, -25.6738)
  line L1664 (-15.175, -25.9738) -> (-15.075, -25.9738)
  line L1665 (-15.075, -25.6738) -> (-15.175, -25.6738)
  line L1666 (-15.925, -25.6738) -> (-15.925, -25.9738)
  line L1667 (-15.925, -25.9738) -> (-15.825, -25.9738)
  line L1668 (-15.825, -25.6738) -> (-15.925, -25.6738)
  line L1669 (-15.825, -25.9738) -> (-15.825, -25.6738)
  line L1670 (-15.675, -25.6738) -> (-15.675, -25.9738)
  line L1671 (-15.575, -25.9738) -> (-15.575, -25.6738)
  line L1672 (-15.575, -25.6738) -> (-15.675, -25.6738)
  line L1673 (-15.675, -25.9738) -> (-15.575, -25.9738)
  line L1674 (-16.425, -25.6738) -> (-16.425, -25.9738)
  line L1675 (-16.425, -25.9738) -> (-16.325, -25.9738)
  line L1676 (-16.325, -25.6738) -> (-16.425, -25.6738)
  line L1677 (-16.325, -25.9738) -> (-16.325, -25.6738)
  line L1678 (-16.175, -25.6738) -> (-16.175, -25.9738)
  line L1679 (-16.075, -25.9738) -> (-16.075, -25.6738)
  line L1680 (-16.075, -25.6738) -> (-16.175, -25.6738)
  line L1681 (-16.175, -25.9738) -> (-16.075, -25.9738)
  line L1682 (-16.925, -25.6738) -> (-16.925, -25.9738)
  line L1683 (-16.925, -25.9738) -> (-16.825, -25.9738)
  line L1684 (-16.825, -25.6738) -> (-16.925, -25.6738)
  line L1685 (-16.825, -25.9738) -> (-16.825, -25.6738)
  line L1686 (-16.675, -25.6738) -> (-16.675, -25.9738)
  line L1687 (-16.575, -25.9738) -> (-16.575, -25.6738)
  line L1688 (-16.675, -25.9738) -> (-16.575, -25.9738)
  line L1689 (-16.575, -25.6738) -> (-16.675, -25.6738)
  line L1690 (-17.075, -25.9738) -> (-17.075, -25.6738)
  line L1691 (-17.175, -25.9738) -> (-17.075, -25.9738)
  line L1692 (-17.075, -25.6738) -> (-17.175, -25.6738)
  line L1693 (-17.175, -25.6738) -> (-17.175, -25.9738)
  line L1694 (-17.325, -25.9738) -> (-17.325, -25.6738)
  line L1695 (-17.425, -25.9738) -> (-17.325, -25.9738)
  line L1696 (-17.325, -25.6738) -> (-17.425, -25.6738)
  line L1697 (-17.425, -25.6738) -> (-17.425, -25.9738)
  line L1698 (-17.675, -25.6738) -> (-17.675, -25.9738)
  line L1699 (-14.175, -25.6738) -> (-14.175, -25.9738)
  line L1700 (-14.175, -25.9738) -> (-14.075, -25.9738)
  line L1701 (-14.075, -25.6738) -> (-14.175, -25.6738)
  line L1702 (-14.075, -25.9738) -> (-14.075, -25.6738)
  line L1703 (-13.925, -25.6738) -> (-13.925, -25.9738)
  line L1704 (-13.825, -25.9738) -> (-13.825, -25.6738)
  line L1705 (-13.925, -25.9738) -> (-13.825, -25.9738)
  line L1706 (-13.825, -25.6738) -> (-13.925, -25.6738)
  line L1707 (3.3, -26.35) -> (3.4, -26.35)
  line L1708 (3.4, -26.35) -> (3.4, -26.05)
  line L1709 (3.4, -26.05) -> (3.3, -26.05)
  line L1710 (3.3, -26.05) -> (3.3, -26.35)
  line L1711 (4.05, -26.05) -> (4.05, -26.35)
  line L1712 (3.8, -26.35) -> (3.9, -26.35)
  line L1713 (3.9, -26.05) -> (3.8, -26.05)
  line L1714 (3.8, -26.05) -> (3.8, -26.35)
  line L1715 (3.675, -25.9738) -> (3.775, -25.9738)
  line L1716 (3.65, -26.05) -> (3.55, -26.05)
  line L1717 (3.925, -25.9738) -> (4.025, -25.9738)
  line L1718 (3.55, -26.35) -> (3.65, -26.35)
  line L1719 (3.55, -26.05) -> (3.55, -26.35)
  line L1720 (3.65, -26.35) -> (3.65, -26.05)
  line L1721 (3.9, -26.35) -> (3.9, -26.05)
  line L1722 (3.425, -25.6738) -> (3.425, -25.9738)
  line L1723 (3.525, -25.6738) -> (3.425, -25.6738)
  line L1724 (3.425, -25.9738) -> (3.525, -25.9738)
  line L1725 (3.525, -25.9738) -> (3.525, -25.6738)
  line L1726 (3.675, -25.6738) -> (3.675, -25.9738)
  line L1727 (3.775, -25.6738) -> (3.675, -25.6738)
  line L1728 (3.775, -25.9738) -> (3.775, -25.6738)
  line L1729 (3.925, -25.6738) -> (3.925, -25.9738)
  line L1730 (4.025, -25.6738) -> (3.925, -25.6738)
  line L1731 (4.025, -25.9738) -> (4.025, -25.6738)
  line L1732 (4.15, -26.35) -> (4.15, -26.05)
  line L1733 (4.05, -26.35) -> (4.15, -26.35)
  line L1734 (4.15, -26.05) -> (4.05, -26.05)
  line L1735 (4.4, -26.05) -> (4.3, -26.05)
  line L1736 (4.3, -26.35) -> (4.4, -26.35)
  line L1737 (4.4, -26.35) -> (4.4, -26.05)
  line L1738 (4.3, -26.05) -> (4.3, -26.35)
  line L1739 (4.525, -25.9738) -> (4.525, -25.6738)
  line L1740 (4.425, -25.9738) -> (4.525, -25.9738)
  line L1741 (4.525, -25.6738) -> (4.425, -25.6738)
  line L1742 (4.425, -25.6738) -> (4.425, -25.9738)
  line L1743 (4.275, -25.9738) -> (4.275, -25.6738)
  line L1744 (4.175, -25.6738) -> (4.175, -25.9738)
  line L1745 (4.275, -25.6738) -> (4.175, -25.6738)
  line L1746 (4.175, -25.9738) -> (4.275, -25.9738)
  line L1747 (4.55, -26.05) -> (4.55, -26.35)
  line L1748 (4.65, -26.05) -> (4.55, -26.05)
  line L1749 (4.55, -26.35) -> (4.65, -26.35)
  line L1750 (4.65, -26.35) -> (4.65, -26.05)
  line L1751 (4.8, -26.35) -> (4.9, -26.35)
  line L1752 (4.9, -26.35) -> (4.9, -26.05)
  line L1753 (4.9, -26.05) -> (4.8, -26.05)
  line L1754 (4.8, -26.05) -> (4.8, -26.35)
  line L1755 (5.025, -25.9738) -> (5.025, -25.6738)
  line L1756 (5.025, -25.6738) -> (4.925, -25.6738)
  line L1757 (4.925, -25.9738) -> (5.025, -25.9738)
  line L1758 (4.925, -25.6738) -> (4.925, -25.9738)
  line L1759 (4.775, -25.9738) -> (4.775, -25.6738)
  line L1760 (4.675, -25.6738) -> (4.675, -25.9738)
  line L1761 (4.775, -25.6738) -> (4.675, -25.6738)
  line L1762 (4.675, -25.9738) -> (4.775, -25.9738)
  line L1763 (5.05, -26.35) -> (5.15, -26.35)
  line L1764 (5.15, -26.35) -> (5.15, -26.05)
  line L1765 (5.15, -26.05) -> (5.05, -26.05)
  line L1766 (5.4, -26.05) -> (5.3, -26.05)
  line L1767 (5.65, -26.05) -> (5.55, -26.05)
  line L1768 (5.05, -26.05) -> (5.05, -26.35)
  line L1769 (5.3, -26.05) -> (5.3, -26.35)
  line L1770 (5.3, -26.35) -> (5.4, -26.35)
  line L1771 (5.4, -26.35) -> (5.4, -26.05)
  line L1772 (5.55, -26.05) -> (5.55, -26.35)
  line L1773 (5.65, -26.35) -> (5.65, -26.05)
  line L1774 (5.55, -26.35) -> (5.65, -26.35)
  line L1775 (5.9, -26.05) -> (5.8, -26.05)
  line L1776 (5.8, -26.05) -> (5.8, -26.35)
  line L1777 (5.9, -26.35) -> (5.9, -26.05)
  line L1778 (5.8, -26.35) -> (5.9, -26.35)
  line L1779 (6.275, -25.9738) -> (6.275, -25.6738)
  line L1780 (6.175, -25.9738) -> (6.275, -25.9738)
  line L1781 (6.275, -25.6738) -> (6.175, -25.6738)
  line L1782 (6.175, -25.6738) -> (6.175, -25.9738)
  line L1783 (6.025, -25.9738) -> (6.025, -25.6738)
  line L1784 (6.025, -25.6738) -> (5.925, -25.6738)
  line L1785 (5.925, -25.9738) -> (6.025, -25.9738)
  line L1786 (5.925, -25.6738) -> (5.925, -25.9738)
  line L1787 (6.675, -25.9738) -> (6.775, -25.9738)
  line L1788 (6.425, -25.9738) -> (6.525, -25.9738)
  line L1789 (6.425, -25.6738) -> (6.425, -25.9738)
  line L1790 (6.525, -25.6738) -> (6.425, -25.6738)
  line L1791 (6.525, -25.9738) -> (6.525, -25.6738)
  line L1792 (6.675, -25.6738) -> (6.675, -25.9738)
  line L1793 (6.775, -25.9738) -> (6.775, -25.6738)
  line L1794 (6.775, -25.6738) -> (6.675, -25.6738)
  line L1795 (6.05, -26.35) -> (6.15, -26.35)
  line L1796 (6.15, -26.35) -> (6.15, -26.05)
  line L1797 (6.15, -26.05) -> (6.05, -26.05)
  line L1798 (6.05, -26.05) -> (6.05, -26.35)
  line L1799 (6.65, -26.05) -> (6.55, -26.05)
  line L1800 (6.4, -26.05) -> (6.3, -26.05)
  line L1801 (6.9, -26.05) -> (6.8, -26.05)
  line L1802 (6.8, -26.35) -> (6.9, -26.35)
  line L1803 (6.9, -26.35) -> (6.9, -26.05)
  line L1804 (6.8, -26.05) -> (6.8, -26.35)
  line L1805 (6.65, -26.35) -> (6.65, -26.05)
  line L1806 (6.55, -26.35) -> (6.65, -26.35)
  line L1807 (6.4, -26.35) -> (6.4, -26.05)
  line L1808 (6.3, -26.35) -> (6.4, -26.35)
  line L1809 (6.3, -26.05) -> (6.3, -26.35)
  line L1810 (6.55, -26.05) -> (6.55, -26.35)
  line L1811 (7.275, -25.9738) -> (7.275, -25.6738)
  line L1812 (7.175, -25.9738) -> (7.275, -25.9738)
  line L1813 (7.275, -25.6738) -> (7.175, -25.6738)
  line L1814 (7.175, -25.6738) -> (7.175, -25.9738)
  line L1815 (6.925, -25.9738) -> (7.025, -25.9738)
  line L1816 (6.925, -25.6738) -> (6.925, -25.9738)
  line L1817 (7.025, -25.6738) -> (6.925, -25.6738)
  line L1818 (7.025, -25.9738) -> (7.025, -25.6738)
  line L1819 (7.4, -26.05) -> (7.3, -26.05)
  line L1820 (7.775, -25.9738) -> (7.775, -25.6738)
  line L1821 (7.675, -25.9738) -> (7.775, -25.9738)
  line L1822 (7.775, -25.6738) -> (7.675, -25.6738)
  line L1823 (7.675, -25.6738) -> (7.675, -25.9738)
  line L1824 (7.425, -25.6738) -> (7.425, -25.9738)
  line L1825 (7.425, -25.9738) -> (7.525, -25.9738)
  line L1826 (7.525, -25.6738) -> (7.425, -25.6738)
  line L1827 (7.525, -25.9738) -> (7.525, -25.6738)
  line L1828 (7.05, -26.35) -> (7.15, -26.35)
  line L1829 (7.15, -26.35) -> (7.15, -26.05)
  line L1830 (7.15, -26.05) -> (7.05, -26.05)
  line L1831 (7.05, -26.05) -> (7.05, -26.35)
  line L1832 (7.9, -26.35) -> (7.9, -26.05)
  line L1833 (7.8, -26.35) -> (7.9, -26.35)
  line L1834 (7.9, -26.05) -> (7.8, -26.05)
  line L1835 (7.8, -26.05) -> (7.8, -26.35)
  line L1836 (7.65, -26.35) -> (7.65, -26.05)
  line L1837 (7.55, -26.35) -> (7.65, -26.35)
  line L1838 (7.65, -26.05) -> (7.55, -26.05)
  line L1839 (7.55, -26.05) -> (7.55, -26.35)
  line L1840 (7.4, -26.35) -> (7.4, -26.05)
  line L1841 (7.3, -26.35) -> (7.4, -26.35)
  line L1842 (7.3, -26.05) -> (7.3, -26.35)
  line L1843 (8.175, -25.9738) -> (8.275, -25.9738)
  line L1844 (7.925, -25.9738) -> (8.025, -25.9738)
  line L1845 (8.025, -25.6738) -> (7.925, -25.6738)
  line L1846 (7.925, -25.6738) -> (7.925, -25.9738)
  line L1847 (8.025, -25.9738) -> (8.025, -25.6738)
  line L1848 (8.175, -25.6738) -> (8.175, -25.9738)
  line L1849 (8.275, -25.9738) -> (8.275, -25.6738)
  line L1850 (8.275, -25.6738) -> (8.175, -25.6738)
  line L1851 (8.05, -26.05) -> (8.05, -26.35)
  line L1852 (8.15, -26.05) -> (8.05, -26.05)
  line L1853 (8.05, -26.35) -> (8.15, -26.35)
  line L1854 (8.15, -26.35) -> (8.15, -26.05)
  line L1855 (8.3, -26.05) -> (8.3, -26.35)
  line L1856 (8.3, -26.35) -> (8.4, -26.35)
  line L1857 (8.4, -26.05) -> (8.3, -26.05)
  line L1858 (8.65, -26.05) -> (8.55, -26.05)
  line L1859 (8.55, -26.35) -> (8.65, -26.35)
  line L1860 (8.65, -26.35) -> (8.65, -26.05)
  line L1861 (8.55, -26.05) -> (8.55, -26.35)
  line L1862 (8.9, -26.05) -> (8.8, -26.05)
  line L1863 (8.4, -26.35) -> (8.4, -26.05)
  line L1864 (8.8, -26.05) -> (8.8, -26.35)
  line L1865 (8.9, -26.35) -> (8.9, -26.05)
  line L1866 (8.8, -26.35) -> (8.9, -26.35)
  line L1867 (8.675, -25.9738) -> (8.775, -25.9738)
  line L1868 (8.925, -25.9738) -> (9.025, -25.9738)
  line L1869 (9.025, -25.9738) -> (9.025, -25.6738)
  line L1870 (9.025, -25.6738) -> (8.925, -25.6738)
  line L1871 (8.925, -25.6738) -> (8.925, -25.9738)
  line L1872 (8.425, -25.9738) -> (8.525, -25.9738)
  line L1873 (8.675, -25.6738) -> (8.675, -25.9738)
  line L1874 (8.775, -25.6738) -> (8.675, -25.6738)
  line L1875 (8.525, -25.9738) -> (8.525, -25.6738)
  line L1876 (8.425, -25.6738) -> (8.425, -25.9738)
  line L1877 (8.525, -25.6738) -> (8.425, -25.6738)
  line L1878 (8.775, -25.9738) -> (8.775, -25.6738)
  line L1879 (9.05, -26.35) -> (9.15, -26.35)
  line L1880 (9.15, -26.35) -> (9.15, -26.05)
  line L1881 (9.15, -26.05) -> (9.05, -26.05)
  line L1882 (9.05, -26.05) -> (9.05, -26.35)
  line L1883 (9.3, -26.35) -> (9.4, -26.35)
  line L1884 (9.4, -26.35) -> (9.4, -26.05)
  line L1885 (9.4, -26.05) -> (9.3, -26.05)
  line L1886 (9.3, -26.05) -> (9.3, -26.35)
  line L1887 (9.55, -26.35) -> (9.65, -26.35)
  line L1888 (9.65, -26.35) -> (9.65, -26.05)
  line L1889 (9.65, -26.05) -> (9.55, -26.05)
  line L1890 (9.9, -26.05) -> (9.8, -26.05)
  line L1891 (9.9, -26.35) -> (9.9, -26.05)
  line L1892 (9.8, -26.35) -> (9.9, -26.35)
  line L1893 (9.8, -26.05) -> (9.8, -26.35)
  line L1894 (9.55, -26.05) -> (9.55, -26.35)
  line L1895 (9.675, -25.9738) -> (9.775, -25.9738)
  line L1896 (9.925, -25.9738) -> (10.025, -25.9738)
  line L1897 (10.025, -25.9738) -> (10.025, -25.6738)
  line L1898 (10.025, -25.6738) -> (9.925, -25.6738)
  line L1899 (9.925, -25.6738) -> (9.925, -25.9738)
  line L1900 (9.775, -25.9738) -> (9.775, -25.6738)
  line L1901 (9.775, -25.6738) -> (9.675, -25.6738)
  line L1902 (9.675, -25.6738) -> (9.675, -25.9738)
  line L1903 (9.425, -25.9738) -> (9.525, -25.9738)
  line L1904 (9.525, -25.9738) -> (9.525, -25.6738)
  line L1905 (9.525, -25.6738) -> (9.425, -25.6738)
  line L1906 (9.175, -25.9738) -> (9.275, -25.9738)
  line L1907 (9.275, -25.9738) -> (9.275, -25.6738)
  line L1908 (9.175, -25.6738) -> (9.175, -25.9738)
  line L1909 (9.275, -25.6738) -> (9.175, -25.6738)
  line L1910 (9.425, -25.6738) -> (9.425, -25.9738)
  line L1911 (5.675, -25.9738) -> (5.775, -25.9738)
  line L1912 (5.425, -25.9738) -> (5.525, -25.9738)
  line L1913 (5.775, -25.9738) -> (5.775, -25.6738)
  line L1914 (5.775, -25.6738) -> (5.675, -25.6738)
  line L1915 (5.675, -25.6738) -> (5.675, -25.9738)
  line L1916 (5.525, -25.9738) -> (5.525, -25.6738)
  line L1917 (5.525, -25.6738) -> (5.425, -25.6738)
  line L1918 (5.425, -25.6738) -> (5.425, -25.9738)
  line L1919 (5.175, -25.9738) -> (5.275, -25.9738)
  line L1920 (5.175, -25.6738) -> (5.175, -25.9738)
  line L1921 (5.275, -25.6738) -> (5.175, -25.6738)
  line L1922 (5.275, -25.9738) -> (5.275, -25.6738)
  line L1923 (10.05, -26.05) -> (10.05, -26.35)
  line L1924 (10.15, -26.05) -> (10.05, -26.05)
  line L1925 (10.05, -26.35) -> (10.15, -26.35)
  line L1926 (10.15, -26.35) -> (10.15, -26.05)
  line L1927 (10.3, -26.05) -> (10.3, -26.35)
  line L1928 (10.3, -26.35) -> (10.4, -26.35)
  line L1929 (10.4, -26.35) -> (10.4, -26.05)
  line L1930 (10.175, -25.9738) -> (10.275, -25.9738)
  line L1931 (10.4, -26.05) -> (10.3, -26.05)
  line L1932 (10.175, -25.6738) -> (10.175, -25.9738)
  line L1933 (10.275, -25.9738) -> (10.275, -25.6738)
  line L1934 (10.275, -25.6738) -> (10.175, -25.6738)
  line L1935 (11.025, -25.9738) -> (11.025, -25.6738)
  line L1936 (10.925, -25.6738) -> (10.925, -25.9738)
  line L1937 (11.025, -25.6738) -> (10.925, -25.6738)
  line L1938 (10.775, -25.9738) -> (10.775, -25.6738)
  line L1939 (10.675, -25.6738) -> (10.675, -25.9738)
  line L1940 (10.775, -25.6738) -> (10.675, -25.6738)
  line L1941 (10.65, -26.05) -> (10.55, -26.05)
  line L1942 (10.425, -25.9738) -> (10.525, -25.9738)
  line L1943 (10.525, -25.9738) -> (10.525, -25.6738)
  line L1944 (10.425, -25.6738) -> (10.425, -25.9738)
  line L1945 (10.525, -25.6738) -> (10.425, -25.6738)
  line L1946 (11.3, -26.35) -> (11.4, -26.35)
  line L1947 (11.4, -26.35) -> (11.4, -26.05)
  line L1948 (11.3, -26.05) -> (11.3, -26.35)
  line L1949 (11.15, -26.35) -> (11.15, -26.05)
  line L1950 (11.15, -26.05) -> (11.05, -26.05)
  line L1951 (11.05, -26.05) -> (11.05, -26.35)
  line L1952 (11.05, -26.35) -> (11.15, -26.35)
  line L1953 (11.525, -25.9738) -> (11.525, -25.6738)
  line L1954 (11.425, -25.9738) -> (11.525, -25.9738)
  line L1955 (11.425, -25.6738) -> (11.425, -25.9738)
  line L1956 (11.525, -25.6738) -> (11.425, -25.6738)
  line L1957 (11.275, -25.9738) -> (11.275, -25.6738)
  line L1958 (11.275, -25.6738) -> (11.175, -25.6738)
  line L1959 (11.175, -25.6738) -> (11.175, -25.9738)
  line L1960 (11.175, -25.9738) -> (11.275, -25.9738)
  line L1961 (11.4, -26.05) -> (11.3, -26.05)
  line L1962 (11.9, -26.35) -> (11.9, -26.05)
  line L1963 (11.8, -26.35) -> (11.9, -26.35)
  line L1964 (11.9, -26.05) -> (11.8, -26.05)
  line L1965 (11.8, -26.05) -> (11.8, -26.35)
  line L1966 (11.65, -26.35) -> (11.65, -26.05)
  line L1967 (11.55, -26.35) -> (11.65, -26.35)
  line L1968 (11.55, -26.05) -> (11.55, -26.35)
  line L1969 (11.65, -26.05) -> (11.55, -26.05)
  line L1970 (13.05, -26.35) -> (13.15, -26.35)
  line L1971 (12.675, -25.9738) -> (12.775, -25.9738)
  line L1972 (12.925, -25.9738) -> (13.025, -25.9738)
  line L1973 (12.675, -25.6738) -> (12.675, -25.9738)
  line L1974 (12.775, -25.6738) -> (12.675, -25.6738)
  line L1975 (12.775, -25.9738) -> (12.775, -25.6738)
  line L1976 (12.025, -25.9738) -> (12.025, -25.6738)
  line L1977 (11.925, -25.9738) -> (12.025, -25.9738)
  line L1978 (12.025, -25.6738) -> (11.925, -25.6738)
  line L1979 (11.925, -25.6738) -> (11.925, -25.9738)
  line L1980 (11.775, -25.9738) -> (11.775, -25.6738)
  line L1981 (11.675, -25.9738) -> (11.775, -25.9738)
  line L1982 (11.675, -25.6738) -> (11.675, -25.9738)
  line L1983 (11.775, -25.6738) -> (11.675, -25.6738)
  line L1984 (10.675, -25.9738) -> (10.775, -25.9738)
  line L1985 (10.925, -25.9738) -> (11.025, -25.9738)
  line L1986 (10.9, -26.35) -> (10.9, -26.05)
  line L1987 (10.8, -26.35) -> (10.9, -26.35)
  line L1988 (10.9, -26.05) -> (10.8, -26.05)
  line L1989 (10.8, -26.05) -> (10.8, -26.35)
  line L1990 (10.65, -26.35) -> (10.65, -26.05)
  line L1991 (10.55, -26.05) -> (10.55, -26.35)
  line L1992 (10.55, -26.35) -> (10.65, -26.35)
  line L1993 (12.175, -25.6738) -> (12.175, -25.9738)
  line L1994 (12.175, -25.9738) -> (12.275, -25.9738)
  line L1995 (12.275, -25.6738) -> (12.175, -25.6738)
  line L1996 (12.275, -25.9738) -> (12.275, -25.6738)
  line L1997 (12.425, -25.6738) -> (12.425, -25.9738)
  line L1998 (12.525, -25.9738) -> (12.525, -25.6738)
  line L1999 (12.525, -25.6738) -> (12.425, -25.6738)
  line L2000 (12.05, -26.05) -> (12.05, -26.35)
  line L2001 (12.15, -26.05) -> (12.05, -26.05)
  line L2002 (12.05, -26.35) -> (12.15, -26.35)
  line L2003 (12.15, -26.35) -> (12.15, -26.05)
  line L2004 (12.3, -26.05) -> (12.3, -26.35)
  line L2005 (12.3, -26.35) -> (12.4, -26.35)
  line L2006 (12.4, -26.35) -> (12.4, -26.05)
  line L2007 (12.4, -26.05) -> (12.3, -26.05)
  line L2008 (12.425, -25.9738) -> (12.525, -25.9738)
  line L2009 (13.175, -25.9738) -> (13.275, -25.9738)
  line L2010 (13.275, -25.6738) -> (13.175, -25.6738)
  line L2011 (13.175, -25.6738) -> (13.175, -25.9738)
  line L2012 (13.025, -25.9738) -> (13.025, -25.6738)
  line L2013 (12.925, -25.6738) -> (12.925, -25.9738)